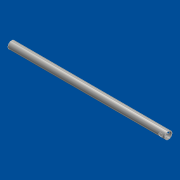
# Autodesk Inventor part: Tubo_conexion
Saved by Autodesk Inventor 2016 (Build 200138000, 138)
## iProperties
Created: 2017-05-13
Part Number: Tubo_conexion
Material: Generic
Document SubType Name: Sheet Metal
Designer: Gian
Density: 1 g/cm^3
Sheet Metal Rule: Default_mm
Appearance: Default
Author: Gian
Autodesk Inventor part; units mm, degrees
ref_plane "YZ Plane" through (0, 0, 0) normal (1, 0, 0) x (0, 1, 0)
ref_plane "XZ Plane" through (0, 0, 0) normal (0, 1, 0) x (-1, 0, 0)
ref_plane "XY Plane" through (0, 0, 0) normal (0, 0, 1) x (1, 0, 0)
sketch "Sketch1" plane through (0, 0, 0) normal (1, 0, 0) x (0, 1, 0)
  circle A0 centre (0, 0) radius 9.525
  dimension "d0" = 19.05
  constraints: 1 centre point
  measures "d0" diameter of A0
sketch "Sketch2" plane through (0, 0, 0) normal (0, 1, 0) x (-1, 0, 0)
  line L0 (0, 0) -> (-398.5, 0)
  dimension "d1" = 398.5
  constraints: 2 end point, 1 horizontal
  measures "d1" distance of L0.start L0.end
sweep "Sweep1" add profiles "Sketch1" path "Sketch2"
sketch "Sketch3" plane through (0, 0, 0) normal (0, 1, 0) x (-1, 0, 0)
  circle A0 centre (-388.1092, 0.0619) radius 5
  dimension "d4" = 10
  constraints: 1 centre point
  measures "d4" diameter of A0
extrude "Cut1" cut sketch "Sketch3" along normal through all both and the other way through all
sketch "Sketch4" plane through (398.5, 0, 0) normal (1, 0, 0) x (0, 0, -1)
  circle A0 centre (0, 0) radius 8.1874
  constraints: 1 centre point
extrude "Cut2" cut sketch "Sketch4" against normal through all
equation "\"d5\" = d4"
equation "\"d7\" = Thickness"
equation "\"BendRadius\" = Thickness"
equation "\"BendReliefWidth\" = Thickness"
equation "\"BendReliefDepth\" = 0.5 * Thickness"
equation "\"CornerReliefSize\" = 4 * Thickness"
equation "\"MinimumRemnant\" = 2 * Thickness"
equation "\"TransitionRadius\" = BendRadius"
equation "\"JacobiRadiusSize\" = BendRadius"
equation "\"GapSize\" = Thickness"
equation "\"Thickness\" = 0.5"
body "Solid1"
